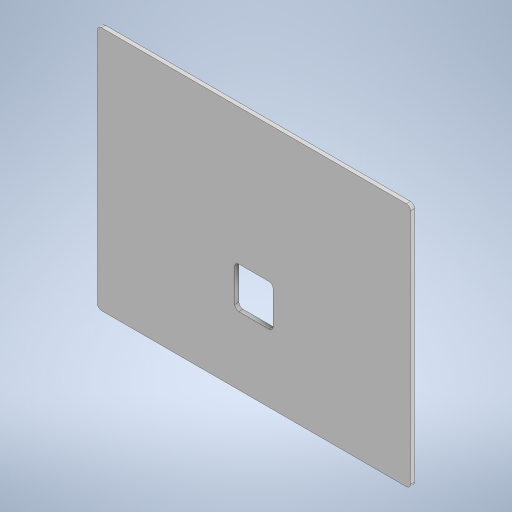
# Autodesk Inventor part: ChamberCamSide
Saved by Autodesk Inventor 2023 (Build 270158000, 158)
## iProperties
Created: 2025-11-21
Part Number: ChamberCamSide
Material: Generic
Document SubType Name: Modeling
Designer: DanAr
Density: 1 g/cm^3
Appearance: Default
Author: DanAr
Autodesk Inventor part; units mm, degrees
ref_plane "YZ Plane" through (0, 0, 0) normal (1, 0, 0) x (0, 1, 0)
ref_plane "XZ Plane" through (0, 0, 0) normal (0, 1, 0) x (-1, 0, 0)
ref_plane "XY Plane" through (0, 0, 0) normal (0, 0, 1) x (1, 0, 0)
sketch "Sketch1" plane through (0, 0, 0) normal (0, 0, 1) x (1, 0, 0)
  line L0 (-14.1, -15.1) -> (14.1, -15.1)
  line L1 (14.1, -15.1) -> (14.1, 15.1)
  line L2 (14.1, 15.1) -> (-14.1, 15.1)
  line L3 (-14.1, 15.1) -> (-14.1, -15.1)
  line L4 (-14.1, -15.1) -> (14.1, 15.1) construction
  line L5 (14.1, -15.1) -> (-14.1, 15.1) construction
  line L6 (-114.9, -114.9) -> (114.9, -114.9)
  line L7 (114.9, -114.9) -> (114.9, 114.9)
  line L8 (114.9, 114.9) -> (-114.9, 114.9)
  line L9 (-114.9, 114.9) -> (-114.9, -114.9)
  line L10 (-114.9, -114.9) -> (114.9, 114.9) construction
  line L11 (114.9, -114.9) -> (-114.9, 114.9) construction
  line L12 (-114.9, -114.9) -> (114.9, -114.9)
  line L13 (114.9, -114.9) -> (114.9, -64.9)
  line L14 (114.9, -64.9) -> (-114.9, -64.9)
  line L15 (-114.9, -64.9) -> (-114.9, -114.9)
  point P0 (0, 0)
  point P1 (-114.9, -64.9)
  dimension "d0" = 28.2
  dimension "d1" = 30.2
  dimension "d2" = 229.8
  dimension "d3" = 229.8
  dimension "d4" = 179.8
  dimension "d9" = 64.9
  dimension "d10" = 114.9
  constraints: 32 end point, 6 parallel, 4 midpoint, 3 horizontal, 3 perpendicular, 1 point on line
  measures "d0" distance of L1.end L2.end
  measures "d1" distance of L0.end L1.end
  measures "d2" distance of L7.end L8.end
  measures "d3" distance of L6.end L7.end
  measures "d4" distance between parallel lines of L8 L14
  measures "d9" distance from line of L14 point (0, 0)
  measures "d10" distance from line of L8 point (0, 0)
extrude "Extrusion1" add sketch "Sketch1" along normal blind 3 contours L9 L8 L7 L14
fillet "Fillet1" radius 3 4 edges at (-14.1, -15.1, 1.5) (-14.1, 15.1, 1.5) (14.1, 15.1, 1.5) (14.1, -15.1, 1.5)
fillet "Fillet2" radius 3 4 edges at (114.9, 114.9, 1.5) (114.9, -64.9, 1.5) (-114.9, -64.9, 1.5) (-114.9, 114.9, 1.5)
body "Solid1"
